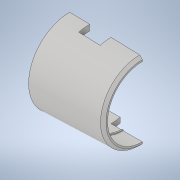
# Autodesk Inventor part: PLASTIC_PART
Saved by Autodesk Inventor 2020.2 (Build 242310000, 310)
## iProperties
Created: 2019-12-16
Part Number: PLASTIC_PART
Material: Generic
Document SubType Name: Modeling
Designer: fabfarm
Density: 1 g/cm^3
Appearance: Default
Author: fabfarm
Autodesk Inventor part; units mm, degrees
ref_plane "YZ Plane" through (0, 0, 0) normal (1, 0, 0) x (0, 1, 0)
ref_plane "XZ Plane" through (0, 0, 0) normal (0, 1, 0) x (-1, 0, 0)
ref_plane "XY Plane" through (0, 0, 0) normal (0, 0, 1) x (1, 0, 0)
sketch "Sketch2" plane through (0, 0, 0) normal (0, 0, 1) x (1, 0, 0)
  line L0 (-31.2032, 0) -> (39.8239, 0) construction
  line L1 (20.125, 19.3) -> (20.125, 21.675)
  line L2 (20.125, 21.675) -> (-20.125, 22.85)
  line L3 (-20.125, 22.85) -> (-20.125, 19.3)
  line L4 (0, 19.3) -> (0, 0) construction
  line L5 (8.775, 19.3) -> (8.775, 18.8)
  line L6 (8.775, 18.8) -> (9.475, 18.8)
  line L7 (9.475, 18.8) -> (9.475, 19.3)
  line L8 (-20.125, 19.3) -> (8.775, 19.3)
  line L9 (9.475, 19.3) -> (20.125, 19.3)
  line L10 (0, 22.2625) -> (0, 19.3) construction
  dimension "d2" = 40.25
  dimension "d34" = 0.5
  dimension "d36" = 0.7
  dimension "d41" = 19.3
  dimension "d45" = 11.35
  dimension "d46" = 22.85
  dimension "d47" = 21.675
  constraints: 22 end point, 5 perpendicular, 4 vertical, 3 horizontal, 2 point on line, 1 collinear, 1 midpoint
  measures "d2" distance of L3.end L1.start
  measures "d34" distance of L5.start L5.end
  measures "d36" distance of L5.end L6.end
  measures "d41" distance between parallel lines of L0 L8
  measures "d45" distance between parallel lines of L5 L1
  measures "d46" distance from line of L2.end L0
  measures "d47" distance from line of L0 L1.end
revolve "Revolution1" add sketch "Sketch2" angle 270 about axis through (-31.2032, 0, 0) along (1, 0, 0)
sketch "Sketch3" plane through (0, 0, 0) normal (0, 1, 0) x (-1, 0, 0)
  line L0 (20.125, 0) -> (20.125, -22.85)
  line L1 (20.125, -22.85) -> (20.125, -22.85)
  line L2 (20.125, -22.85) -> (20.125, 0)
  line L3 (20.125, 0) -> (20.125, 0)
  line L4 (-20.125, -19.3) -> (-20.125, -21.675) projected
  line L5 (-20.125, -21.675) -> (-20.125, 0)
  line L6 (-2.725, -5) -> (-2.725, 0)
  line L7 (9.125, -5) -> (-2.725, -5)
  line L8 (-20.125, -21.675) -> (20.125, -22.85) projected
  line L9 (20.125, -22.85) -> (-20.125, -21.675)
  line L10 (-2.725, 0) -> (-20.125, 0)
  line L11 (20.125, 0) -> (9.125, 0)
  line L12 (9.125, 0) -> (9.125, -5)
  dimension "d21" = 11
  dimension "d23" = 5
  dimension "d43" = 11.85
  constraints: 22 end point, 3 collinear, 3 horizontal, 3 vertical, 1 perpendicular
  measures "d21" distance of L2.end L11.end
  measures "d23" distance of L6.start L6.end
  measures "d43" distance of L7.start L6.start
extrude "Extrusion1" cut sketch "Sketch3" against normal blind 200
sketch "Sketch4" plane through (0, 0, 0) normal (0, 1, 0) x (-1, 0, 0)
  line L0 (-20.125, 0) -> (20.125, 0) projected
  line L1 (9.125, 0) -> (-2.725, 0)
  line L2 (-2.725, 0) -> (-2.725, 6)
  line L3 (-2.725, 6) -> (9.125, 6)
  line L4 (9.125, 6) -> (9.125, 0)
  line L5 (20.125, 22.85) -> (20.125, 0) projected
  line L6 (-20.125, 21.675) -> (-20.125, 0) projected
  point P0 (-2.725, 0)
  dimension "d24" = 6
  dimension "d25" = 11
  dimension "d44" = 11.85
  constraints: 8 end point, 2 parallel, 1 horizontal, 1 perpendicular, 1 point on line
  measures "d24" distance of L1.end L2.end
  measures "d25" distance between parallel lines of L5 L4
  measures "d44" distance of L2.end L3.end
extrude "Extrusion2" cut sketch "Sketch4" along normal blind 200
chamfer "Chamfer1" distance 1.5 angle 45 1 edges at (20.125, 0, 21.675)
body "Solid1"
